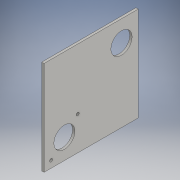
# Autodesk Inventor part: GearboxPlate1
Saved by Autodesk Inventor 2016 (Build 200138000, 138)
## iProperties
Created: 2017-01-21
Part Number: GearboxPlate1
Material: Generic
Document SubType Name: Modeling
Designer: Nick
Density: 1 g/cm^3
Appearance: Default
Author: Nick
Autodesk Inventor part; units mm, degrees
ref_plane "YZ Plane" through (0, 0, 0) normal (1, 0, 0) x (0, 1, 0)
ref_plane "XZ Plane" through (0, 0, 0) normal (0, 1, 0) x (-1, 0, 0)
ref_plane "XY Plane" through (0, 0, 0) normal (0, 0, 1) x (1, 0, 0)
sketch "Sketch1" plane through (0, 0, 0) normal (0, 0, 1) x (1, 0, 0)
  line L0 (-59.4683, 37.7867) -> (67.5317, 37.7867)
  line L1 (67.5317, 37.7867) -> (67.5317, -89.2133)
  line L2 (67.5317, -89.2133) -> (-59.4683, -89.2133)
  line L3 (-59.4683, -89.2133) -> (-59.4683, 37.7867)
  line L4 (-59.4683, -89.2133) -> (-18.4383, -89.2133)
  line L5 (-60.4499, -32.9669) -> (-59.4683, -89.2133)
  line L6 (-53.1183, 31.4367) -> (-11.1067, 31.4367)
  line L7 (-11.1067, 31.4367) -> (-11.1067, -10.5749)
  line L8 (-11.1067, -10.5749) -> (-53.1183, -10.5749)
  line L9 (-53.1183, -10.5749) -> (-53.1183, 31.4367)
  circle A0 centre (39.3264, -66.5565) radius 14.3002
  circle A1 centre (-32.1633, 10.3801) radius 14.1986
  circle A2 centre (-14.1547, -7.5269) radius 2.0193
  circle A3 centre (-50.0703, 28.3887) radius 2.0193
  point P0 (0, 0)
  dimension "d0" = 127
  dimension "d1" = 127
  dimension "d8" = 42.0116
  dimension "d9" = 42.0116
  dimension "d10" = 3.048
  dimension "d13" = 3.048
  dimension "d14" = 6.35
  dimension "d15" = 6.35
  dimension "d16" = 3.048
  dimension "d17" = 3.048
  dimension "d18" = 20.955
  dimension "d19" = 20.955
  dimension "d21" = 28.6004
  dimension "d23" = 105.0239
  dimension "d26" = 28.3972
  dimension "d27" = 4.0386
  dimension "d28" = 4.0386
  constraints: 20 end point, 4 centre point, 4 parallel, 3 coincident, 3 horizontal, 2 perpendicular
  measures "d0" distance of L0.start L0.end
  measures "d1" distance of L0.end L1.end
  measures "d8" distance of L6.end L7.end
  measures "d9" distance of L7.end L8.end
  measures "d10" distance from line of L6 point (-50.07, 28.389)
  measures "d13" distance from line of L8 point (-14.155, -7.527)
  measures "d14" distance between parallel lines of L6 L0
  measures "d15" distance between parallel lines of L3 L9
  measures "d16" distance from line of L7 point (-14.155, -7.527)
  measures "d17" distance from line of L9 point (-50.07, 28.389)
  measures "d18" distance from line of L8 point (-32.163, 10.38)
  measures "d19" distance from line of L9 point (-32.163, 10.38)
  measures "d21" diameter of A0
  measures "d23" distance of A0.centre point (-32.163, 10.38)
  measures "d26" diameter of A1
  measures "d27" diameter of A3
  measures "d28" diameter of A2
extrude "Extrusion1" add sketch "Sketch1" along normal blind 3.175 contours L0 L1 L2 L3 | L6 L7 L8 L9
body "Solid1"
